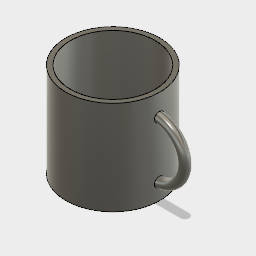
水杯 (Autodesk Fusion 360 design; units mm, degrees)
Autodesk Fusion 360 part; units mm, degrees
sketch "草图1" plane through (0, 0, 0) normal (0, 1, 0) x (1, 0, 0)
  circle A0 centre (0, 0) radius 10
extrude "拉伸1" add sketch "草图1" along normal blind 20 makes body 1
cylinder "圆柱体基本要素1" add diameter 18 height 20 placed x (1, 0, 0) y (0, 0, -1) z (0, 1, 0) at (0, 0, 40) separate body makes body 2
torus "圆环体基本要素1" add centre line diameter 12 section diameter 2 placed x (1, 0, 0) y (0, 0, -1) z (0, 1, 0) at (30, 0, -35) separate body makes body 3
move_body "MoveFace1" bodies 3 to x (1, 0, 0) y (0, 0, 1) z (0, -1, 0) at (0, -35, -35) on bodies 3
move_body "MoveFace7" bodies 3 to x (1, 0, 0) y (0, 1, 0) z (0, 0, 1) at (0, 10.0841, 35.1004) on bodies 3
move_body "移动1" bodies 2 to x (1, 0, 0) y (0, 1, 0) z (0, 0, 1) at (-74.6356, 6.0443, -15.2315)
move_body "MoveFace8" bodies 3 to x (1, 0, 0) y (0, 1, 0) z (0, 0, 1) at (-20.5561, -0.5818, 0) on bodies 3
combine "合并1" operation add target body 1 tool bodies 3
move_body "对齐1" bodies 2 to x (1, 0, 0) y (0, 1, 0) z (0, 0, 1) at (74.6356, -6.0443, -24.7685)
sketch "草图4" plane through (0, 0, 0) normal (0, 1, 0) x (1, 0, 0)
  line L0 (-19, 21) -> (-19, 13)
  line L1 (-19, 13) -> (-14, 21)
  line L2 (-14, 21) -> (-19, 21)
move_face "偏移面1" offset -2 1 faces at (-5.1676, 0, -0.3267) on bodies 2
combine "合并2" operation cut target body 1 tool bodies 2
moveface "MoveFace5" [rolled back]
moveface "MoveFace6" [rolled back]
moveface "MoveFace2" [rolled back]
moveface "MoveFace3" [rolled back]
moveface "MoveFace4" [rolled back]
